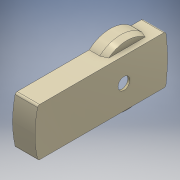
# Autodesk Inventor part: ET9
Saved by Autodesk Inventor 2016 (Build 200138000, 138)
## iProperties
Created: 2016-03-20
Part Number: ET9
Material: Genérico
Document SubType Name: Modeling
Designer: Usuario1
Density: 1 g/cm^3
Appearance: Valor por defecto
Author: Usuario1
Autodesk Inventor part; units mm, degrees
ref_plane "YZ Plane" through (0, 0, 0) normal (1, 0, 0) x (0, 1, 0)
ref_plane "XZ Plane" through (0, 0, 0) normal (0, 1, 0) x (-1, 0, 0)
ref_plane "XY Plane" through (0, 0, 0) normal (0, 0, 1) x (1, 0, 0)
sketch "Boceto1" plane through (0, 0, 0) normal (1, 0, 0) x (0, 1, 0)
  arc A0 (0.0357, 0.1637) -> (0.0357, -3.0114) centre (6.9261, -1.4239) ccw
  arc A1 (0.0357, -3.0114) -> (0.1818, -3.1278) centre (0.1818, -2.9778) ccw
  arc A2 (0.1818, 0.28) -> (0.0357, 0.1637) centre (0.1818, 0.13) ccw
  arc A3 (9.1854, -2.9976) -> (9.1854, 0.1498) centre (-2.6213, -1.4239) ccw
  arc A4 (9.0368, -3.1278) -> (9.1854, -2.9976) centre (9.0368, -2.9778) ccw
  arc A5 (9.1854, 0.1498) -> (9.0368, 0.28) centre (9.0368, 0.13) ccw
  line L0 (9.0368, 0.28) -> (8.2953, 0.28)
  line L1 (9.0368, -3.1278) -> (8.2953, -3.1278)
  line L2 (5.3121, 0.28) -> (0.1818, 0.28)
  line L3 (0.1818, -3.1278) -> (5.3121, -3.1278)
  arc A6 (8.2953, 0.28) -> (5.3121, 0.28) centre (6.8037, -1.4239) ccw
  arc A7 (5.3121, -3.1278) -> (8.2953, -3.1278) centre (6.8037, -1.4239) ccw
  arc A8 (9.0368, -2.9778) -> (9.0368, 0.13) centre (-2.6213, -1.4239) ccw
  line L4 (9.0368, -2.9778) -> (8.2378, -2.9778)
  arc A9 (5.3695, -2.9778) -> (8.2378, -2.9778) centre (6.8037, -1.4239) ccw
  line L5 (5.3695, -2.9778) -> (0.1818, -2.9778)
  arc A10 (0.1818, 0.13) -> (0.1818, -2.9778) centre (6.9261, -1.4239) ccw
  line L6 (0.1818, 0.13) -> (5.3695, 0.13)
  arc A11 (8.2378, 0.13) -> (5.3695, 0.13) centre (6.8037, -1.4239) ccw
  line L7 (8.2378, 0.13) -> (9.0368, 0.13)
  point P0 (0, 0)
  dimension "d0" = 0.15
  constraints: 24 point on circle, 16 end point, 12 centre point, 7 other
  measures "d0" radial gap between concentric circles of A3 A8
extrude "Extrusión1" add sketch "Boceto1" along normal blind 0.45
sketch "Boceto2" plane through (0.45, 0, 0) normal (1, 0, 0) x (0, 0, -1)
  line L0 (2.9778, 9.0368) -> (2.9778, 8.2378) projected
  arc A0 (2.9778, 5.3695) -> (2.9778, 8.2378) centre (1.4239, 6.8037) ccw projected
  line L1 (2.9778, 5.3695) -> (2.9778, 0.1818) projected
  arc A1 (-0.13, 0.1818) -> (2.9778, 0.1818) centre (1.4239, 6.9261) ccw projected
  line L2 (-0.13, 0.1818) -> (-0.13, 5.3695) projected
  arc A2 (-0.13, 8.2378) -> (-0.13, 5.3695) centre (1.4239, 6.8037) ccw projected
  line L3 (-0.13, 8.2378) -> (-0.13, 9.0368) projected
  arc A3 (2.9778, 9.0368) -> (-0.13, 9.0368) centre (1.4239, -2.6213) ccw projected
  arc A4 (-0.1637, 0.0357) -> (3.0114, 0.0357) centre (1.4239, 6.9261) ccw projected
  arc A5 (3.0114, 0.0357) -> (3.1278, 0.1818) centre (2.9778, 0.1818) ccw projected
  line L4 (3.1278, 0.1818) -> (3.1278, 5.3121) projected
  arc A6 (3.1278, 5.3121) -> (3.1278, 8.2953) centre (1.4239, 6.8037) ccw projected
  line L5 (3.1278, 8.2953) -> (3.1278, 9.0368) projected
  arc A7 (3.1278, 9.0368) -> (2.9976, 9.1854) centre (2.9778, 9.0368) ccw projected
  arc A8 (2.9976, 9.1854) -> (-0.1498, 9.1854) centre (1.4239, -2.6213) ccw projected
  arc A9 (-0.1498, 9.1854) -> (-0.28, 9.0368) centre (-0.13, 9.0368) ccw projected
  line L6 (-0.28, 9.0368) -> (-0.28, 8.2953) projected
  arc A10 (-0.28, 8.2953) -> (-0.28, 5.3121) centre (1.4239, 6.8037) ccw projected
  line L7 (-0.28, 5.3121) -> (-0.28, 0.1818) projected
  arc A11 (-0.28, 0.1818) -> (-0.1637, 0.0357) centre (-0.13, 0.1818) ccw projected
  line L8 (-0.13, 8.2378) -> (-0.13, 5.3695)
  arc A12 (2.9778, 5.3695) -> (2.9778, 8.2378) centre (1.4239, 6.8037) ccw projected
  line L9 (2.9778, 5.3695) -> (2.9778, 8.2378)
  point P0 (0, 0)
  constraints: 4 end point, 2 vertical
extrude "Extrusión2" add sketch "Boceto2" against normal blind 0.35 contours A0 L9 | L8 A2
chamfer "Chaflán1" distance 0.45 angle 15 1 edges at (0.45, 6.8037, -3.6884) measured on face at (0.35, 6.8037, -3.6884)
chamfer "Chaflán2" distance 0.45 angle 15 1 edges at (0.45, 6.8037, 0.8406) measured on face at (0.35, 6.8037, 0.8406)
sketch "Boceto3" plane through (0.45, 0, 0) normal (1, 0, 0) x (0, 0, -1)
  line L0 (-0.28, 0.1818) -> (-0.28, 5.5024) projected
  arc A0 (-0.28, 0.1818) -> (-0.1637, 0.0357) centre (-0.13, 0.1818) ccw projected
  arc A1 (-0.1637, 0.0357) -> (3.0114, 0.0357) centre (1.4239, 6.9261) ccw projected
  arc A2 (3.0114, 0.0357) -> (3.1278, 0.1818) centre (2.9778, 0.1818) ccw projected
  line L1 (3.1278, 0.1818) -> (3.1278, 5.5024) projected
  arc A3 (3.1278, 5.5024) -> (3.1278, 8.1049) centre (1.4239, 6.8037) ccw projected
  line L2 (3.1278, 9.0368) -> (3.1278, 8.1049) projected
  arc A4 (3.1278, 9.0368) -> (2.9976, 9.1854) centre (2.9778, 9.0368) ccw projected
  arc A5 (2.9976, 9.1854) -> (-0.1498, 9.1854) centre (1.4239, -2.6213) ccw projected
  arc A6 (-0.1498, 9.1854) -> (-0.28, 9.0368) centre (-0.13, 9.0368) ccw projected
  line L3 (-0.28, 9.0368) -> (-0.28, 8.1049) projected
  arc A7 (-0.28, 8.1049) -> (-0.28, 5.5024) centre (1.4239, 6.8037) ccw projected
  line L4 (2.9778, 9.0368) -> (2.9778, 0.1818) projected
  arc A8 (-0.13, 0.1818) -> (2.9778, 0.1818) centre (1.4239, 6.9261) ccw projected
  line L5 (-0.13, 0.1818) -> (-0.13, 9.0368) projected
  arc A9 (2.9778, 9.0368) -> (-0.13, 9.0368) centre (1.4239, -2.6213) ccw projected
  line L6 (-0.28, 8.1049) -> (-0.28, 5.5024)
  line L7 (3.1278, 8.1049) -> (3.1278, 5.5024)
  point P0 (0, 0)
  constraints: 4 end point, 1 parallel, 1 vertical
extrude "Extrusión3" add sketch "Boceto3" along normal blind 0.4 contours L0 L6 L3 A6 A5 A4 L2 L7 L1 A2 A1 A0
sketch "Boceto4" plane through (0.85, 0, 0) normal (1, 0, 0) x (0, 0, -1)
  arc A0 (-0.13, 0.1818) -> (2.9778, 0.1818) centre (1.4239, 6.9261) ccw projected
  line L0 (-0.13, 0.1818) -> (-0.13, 9.0368) projected
  arc A1 (2.9778, 9.0368) -> (-0.13, 9.0368) centre (1.4239, -2.6213) ccw projected
  line L1 (2.9778, 9.0368) -> (2.9778, 0.1818) projected
  line L2 (-0.28, 9.0368) -> (-0.28, 0.1818) projected
  arc A2 (-0.28, 0.1818) -> (-0.1637, 0.0357) centre (-0.13, 0.1818) ccw projected
  arc A3 (-0.1637, 0.0357) -> (3.0114, 0.0357) centre (1.4239, 6.9261) ccw projected
  arc A4 (3.0114, 0.0357) -> (3.1278, 0.1818) centre (2.9778, 0.1818) ccw projected
  line L3 (3.1278, 0.1818) -> (3.1278, 9.0368) projected
  arc A5 (3.1278, 9.0368) -> (2.9976, 9.1854) centre (2.9778, 9.0368) ccw projected
  arc A6 (2.9976, 9.1854) -> (-0.1498, 9.1854) centre (1.4239, -2.6213) ccw projected
  arc A7 (-0.1498, 9.1854) -> (-0.28, 9.0368) centre (-0.13, 9.0368) ccw projected
  point P0 (0, 0)
extrude "Extrusión4" add sketch "Boceto4" against normal blind 0.15 contours L0 A1 L1 A0
sketch "Boceto5" plane through (0, 0, 0) normal (-1, 0, 0) x (0, 0, 1)
  line L0 (-2.9778, 8.2378) -> (-2.9778, 9.0368) projected
  arc A0 (0.13, 9.0368) -> (-2.9778, 9.0368) centre (-1.4239, -2.6213) ccw projected
  line L1 (0.13, 9.0368) -> (0.13, 8.2378) projected
  arc A1 (0.13, 5.3695) -> (0.13, 8.2378) centre (-1.4239, 6.8037) ccw projected
  line L2 (0.13, 5.3695) -> (0.13, 0.1818) projected
  arc A2 (-2.9778, 0.1818) -> (0.13, 0.1818) centre (-1.4239, 6.9261) ccw projected
  line L3 (-2.9778, 0.1818) -> (-2.9778, 5.3695) projected
  arc A3 (-2.9778, 8.2378) -> (-2.9778, 5.3695) centre (-1.4239, 6.8037) ccw projected
  arc A4 (-3.0114, 0.0357) -> (0.1637, 0.0357) centre (-1.4239, 6.9261) ccw projected
  arc A5 (0.1637, 0.0357) -> (0.28, 0.1818) centre (0.13, 0.1818) ccw projected
  line L4 (0.28, 5.3121) -> (0.28, 0.1818) projected
  arc A6 (0.28, 5.3121) -> (0.28, 8.2953) centre (-1.4239, 6.8037) ccw projected
  line L5 (0.28, 9.0368) -> (0.28, 8.2953) projected
  arc A7 (0.28, 9.0368) -> (0.1498, 9.1854) centre (0.13, 9.0368) ccw projected
  arc A8 (0.1498, 9.1854) -> (-2.9976, 9.1854) centre (-1.4239, -2.6213) ccw projected
  arc A9 (-2.9976, 9.1854) -> (-3.1278, 9.0368) centre (-2.9778, 9.0368) ccw projected
  line L6 (-3.1278, 8.2953) -> (-3.1278, 9.0368) projected
  arc A10 (-3.1278, 8.2953) -> (-3.1278, 5.3121) centre (-1.4239, 6.8037) ccw projected
  line L7 (-3.1278, 0.1818) -> (-3.1278, 5.3121) projected
  arc A11 (-3.1278, 0.1818) -> (-3.0114, 0.0357) centre (-2.9778, 0.1818) ccw projected
  arc A12 (-3.0114, 0.0357) -> (0.1637, 0.0357) centre (-1.4239, 6.9261) ccw
  arc A13 (0.1637, 0.0357) -> (0.28, 0.1818) centre (0.13, 0.1818) ccw
  arc A14 (-3.1278, 0.1818) -> (-3.0114, 0.0357) centre (-2.9778, 0.1818) ccw
  circle A15 centre (-1.4239, 6.8037) radius 2.0393
  circle A16 centre (-2.9794, 4.0685) radius 0.092
  arc A17 (0.1498, 9.1854) -> (-2.9976, 9.1854) centre (-1.4239, -2.6213) ccw
  arc A18 (0.28, 9.0368) -> (0.1498, 9.1854) centre (0.13, 9.0368) ccw
  arc A19 (-2.9976, 9.1854) -> (-3.1278, 9.0368) centre (-2.9778, 9.0368) ccw
  line L8 (-3.1278, 3.94) -> (-2.9678, 3.94)
  arc A20 (-2.9678, 3.94) -> (-2.8478, 4.06) centre (-2.9678, 4.06) ccw
  line L9 (-2.8478, 4.06) -> (-2.8478, 4.0786)
  arc A21 (-2.8478, 4.0786) -> (-2.9678, 4.1986) centre (-2.9678, 4.0786) ccw
  line L10 (-2.9678, 4.1986) -> (-3.1278, 4.1986)
  circle A22 centre (-2.9778, 9.0368) radius 0.092
  line L11 (-3.1278, 8.9082) -> (-2.9678, 8.9082)
  line L12 (-2.8478, 9.2044) -> (-2.8478, 9.0282)
  arc A23 (-2.9678, 8.9082) -> (-2.8478, 9.0282) centre (-2.9678, 9.0282) ccw
  circle A24 centre (-2.9778, 0.1818) radius 0.092
  line L13 (-3.1278, 0.3104) -> (-2.9678, 0.3104)
  line L14 (-2.8478, 0) -> (-2.8478, 0.1904)
  arc A25 (-2.8478, 0.1904) -> (-2.9678, 0.3104) centre (-2.9678, 0.1904) ccw
  circle A26 centre (0.1317, 4.0685) radius 0.092
  line L15 (0.28, 3.94) -> (0.12, 3.94)
  arc A27 (0, 4.06) -> (0.12, 3.94) centre (0.12, 4.06) ccw
  line L16 (0, 4.06) -> (0, 4.0786)
  arc A28 (0.12, 4.1986) -> (0, 4.0786) centre (0.12, 4.0786) ccw
  line L17 (0.12, 4.1986) -> (0.28, 4.1986)
  circle A29 centre (0.13, 9.0368) radius 0.092
  line L18 (0.28, 8.9082) -> (0.12, 8.9082)
  line L19 (0, 9.2044) -> (0, 9.0282)
  arc A30 (0, 9.0282) -> (0.12, 8.9082) centre (0.12, 9.0282) ccw
  circle A31 centre (0.13, 0.1818) radius 0.092
  line L20 (0.28, 0.3104) -> (0.12, 0.3104)
  line L21 (0, 0) -> (0, 0.1904)
  arc A32 (0.12, 0.3104) -> (0, 0.1904) centre (0.12, 0.1904) ccw
  line L22 (-3.1278, 9.0368) -> (-3.1278, 8.2953)
  line L23 (0.28, 9.0368) -> (0.28, 8.2953)
  line L24 (-3.1278, 5.3121) -> (-3.1278, 0.1818)
  line L25 (0.28, 0.1818) -> (0.28, 5.3121)
  arc A33 (-3.1278, 8.2953) -> (-3.1278, 5.3121) centre (-1.4239, 6.8037) ccw
  arc A34 (0.28, 5.3121) -> (0.28, 8.2953) centre (-1.4239, 6.8037) ccw
  point P0 (0, 0)
  constraints: 36 end point, 36 point on circle, 23 centre point, 8 point on line
extrude "Extrusión5" add sketch "Boceto5" against normal blind 0.75 contours L11 L6 A9 A8 L12 A0 A22 L0 | L0 A22 A0 L12 A23 L11 | A22 A0 L0 | L0 A0 A22 | L10 A21 L9 A20 L8 L3 A16 | L3 A16 L8 L7 L10 | A16 L3 | L3 A16 | L19 A8 A7 L5 L18 L1 A29 A0 | A0 A29 L1 L18 A30 L19 | L13 L3 A24 A2 L14 A4 A11 L7 | A29 L1 A0 | A0 L1 A29 | L13 A25 L14 A2 A24 L3 | A24 A2 L3 | L3 A2 A24 | L21 A2 A31 L2 L20 L4 A5 A4 | L21 A32 L20 L2 A31 A2 | L17 L4 L15 L2 A26 | L2 A26 L15 A27 L16 A28 L17 | A31 L2 A2 | A2 L2 A31 | A26 L2 | L2 A26
sketch "Boceto6" plane through (0.1, 0, 0) normal (-1, 0, 0) x (0, 0, 1)
  line L0 (-2.9778, 5.3695) -> (-2.9778, 8.2378) projected
  arc A0 (-2.9778, 8.2378) -> (-2.9778, 5.3695) centre (-1.4239, 6.8037) ccw projected
  line L1 (0.13, 8.2378) -> (0.13, 5.3695) projected
  arc A1 (0.13, 5.3695) -> (0.13, 8.2378) centre (-1.4239, 6.8037) ccw projected
  point P0 (0, 0)
extrude "Extrusión6" add sketch "Boceto6" along normal blind 0.1
sketch "Boceto7" plane through (0, 0, 0) normal (-1, 0, 0) x (0, 0, 1)
  arc A0 (-2.8478, 0.1532) -> (0, 0.1532) centre (-1.4239, 6.9261) ccw projected
  line L0 (-2.8478, 0.1532) -> (-2.8478, 0.1904) projected
  arc A1 (-2.8478, 0.1904) -> (-2.9678, 0.3104) centre (-2.9678, 0.1904) ccw projected
  line L1 (-2.9678, 0.3104) -> (-2.9778, 0.3104) projected
  line L2 (-2.9778, 0.3104) -> (-2.9778, 3.94) projected
  line L3 (-2.9778, 3.94) -> (-2.9678, 3.94) projected
  arc A2 (-2.9678, 3.94) -> (-2.8478, 4.06) centre (-2.9678, 4.06) ccw projected
  line L4 (-2.8478, 4.06) -> (-2.8478, 4.0786) projected
  arc A3 (-2.8478, 4.0786) -> (-2.9678, 4.1986) centre (-2.9678, 4.0786) ccw projected
  line L5 (-2.9678, 4.1986) -> (-2.9778, 4.1986) projected
  line L6 (-2.9778, 4.1986) -> (-2.9778, 8.9082) projected
  line L7 (-2.9778, 8.9082) -> (-2.9678, 8.9082) projected
  arc A4 (-2.9678, 8.9082) -> (-2.8478, 9.0282) centre (-2.9678, 9.0282) ccw projected
  line L8 (-2.8478, 9.0282) -> (-2.8478, 9.0533) projected
  arc A5 (0, 9.0533) -> (-2.8478, 9.0533) centre (-1.4239, -2.6213) ccw projected
  line L9 (0, 9.0533) -> (0, 9.0282) projected
  arc A6 (0, 9.0282) -> (0.12, 8.9082) centre (0.12, 9.0282) ccw projected
  line L10 (0.12, 8.9082) -> (0.13, 8.9082) projected
  line L11 (0.13, 8.9082) -> (0.13, 4.1986) projected
  line L12 (0.13, 4.1986) -> (0.12, 4.1986) projected
  arc A7 (0.12, 4.1986) -> (0, 4.0786) centre (0.12, 4.0786) ccw projected
  line L13 (0, 4.0786) -> (0, 4.06) projected
  arc A8 (0, 4.06) -> (0.12, 3.94) centre (0.12, 4.06) ccw projected
  line L14 (0.12, 3.94) -> (0.13, 3.94) projected
  line L15 (0.13, 3.94) -> (0.13, 0.3104) projected
  line L16 (0.13, 0.3104) -> (0.12, 0.3104) projected
  arc A9 (0.12, 0.3104) -> (0, 0.1904) centre (0.12, 0.1904) ccw projected
  line L17 (0, 0.1904) -> (0, 0.1532) projected
  arc A10 (-3.0114, 0.0357) -> (0.1637, 0.0357) centre (-1.4239, 6.9261) ccw projected
  arc A11 (0.1637, 0.0357) -> (0.28, 0.1818) centre (0.13, 0.1818) ccw projected
  line L18 (0.28, 5.3121) -> (0.28, 0.1818) projected
  arc A12 (0.28, 5.3121) -> (0.28, 8.2953) centre (-1.4239, 6.8037) ccw projected
  line L19 (0.28, 9.0368) -> (0.28, 8.2953) projected
  arc A13 (0.28, 9.0368) -> (0.1498, 9.1854) centre (0.13, 9.0368) ccw projected
  arc A14 (0.1498, 9.1854) -> (-2.9976, 9.1854) centre (-1.4239, -2.6213) ccw projected
  arc A15 (-2.9976, 9.1854) -> (-3.1278, 9.0368) centre (-2.9778, 9.0368) ccw projected
  line L20 (-3.1278, 8.2953) -> (-3.1278, 9.0368) projected
  arc A16 (-3.1278, 8.2953) -> (-3.1278, 5.3121) centre (-1.4239, 6.8037) ccw projected
  line L21 (-3.1278, 0.1818) -> (-3.1278, 5.3121) projected
  arc A17 (-3.1278, 0.1818) -> (-3.0114, 0.0357) centre (-2.9778, 0.1818) ccw projected
  line L22 (0.28, 8.2953) -> (0.28, 5.3121)
  line L23 (-3.1278, 8.2953) -> (-3.1278, 9.0368) projected
  line L24 (-3.1278, 5.3121) -> (-3.1278, 8.2953)
  point P0 (0, 0)
  constraints: 4 end point, 1 collinear, 1 vertical
extrude "Extrusión7" add sketch "Boceto7" along normal blind 0.75 contours A17 L21 L24 L20 A15 A14 A13 L19 L22 L18 A11 A10
sketch "Boceto8" plane through (0, 0, 0) normal (-1, 0, 0) x (0, 0, 1)
  arc A0 (-3.1278, 8.1049) -> (-3.1278, 5.5024) centre (-1.4239, 6.8037) ccw projected
  arc A1 (-3.1278, 8.2953) -> (-3.1278, 5.3121) centre (-1.4239, 6.8037) ccw projected
  arc A2 (0.28, 5.5024) -> (0.28, 8.1049) centre (-1.4239, 6.8037) ccw projected
  arc A3 (0.28, 5.3121) -> (0.28, 8.2953) centre (-1.4239, 6.8037) ccw projected
  line L0 (-3.1278, 9.0368) -> (-3.1278, 0.1818) projected
  line L1 (0.28, 0.1818) -> (0.28, 9.0368) projected
  point P0 (0, 0)
extrude "Extrusión8" add sketch "Boceto8" along normal blind 0.75 contours A0 L0 A1 | A2 L1 A3
sketch "Boceto9" plane through (-0.75, 0, 0) normal (-1, 0, 0) x (0, 0, 1)
  arc A0 (0.28, 5.5024) -> (0.28, 8.1049) centre (-1.4239, 6.8037) ccw projected
  line L0 (0.28, 5.5024) -> (0.13, 5.5024)
  line L1 (0.13, 8.9082) -> (0.13, 4.1986) projected
  line L2 (0.28, 5.5024) -> (0.13, 5.5024)
  line L3 (-3.1278, 5.3121) -> (-3.1278, 0.1818) projected
  arc A1 (-3.1278, 0.1818) -> (-3.0114, 0.0357) centre (-2.9778, 0.1818) ccw projected
  arc A2 (-3.0114, 0.0357) -> (0.1637, 0.0357) centre (-1.4239, 6.9261) ccw projected
  arc A3 (0.1637, 0.0357) -> (0.28, 0.1818) centre (0.13, 0.1818) ccw projected
  line L4 (0.28, 0.1818) -> (0.28, 5.3121) projected
  arc A4 (0.28, 5.3121) -> (0.28, 8.2953) centre (-1.4239, 6.8037) ccw projected
  line L5 (0.28, 8.2953) -> (0.28, 9.0368) projected
  arc A5 (0.28, 9.0368) -> (0.1498, 9.1854) centre (0.13, 9.0368) ccw projected
  arc A6 (0.1498, 9.1854) -> (-2.9976, 9.1854) centre (-1.4239, -2.6213) ccw projected
  arc A7 (-2.9976, 9.1854) -> (-3.1278, 9.0368) centre (-2.9778, 9.0368) ccw projected
  line L6 (-3.1278, 9.0368) -> (-3.1278, 8.2953) projected
  arc A8 (-3.1278, 8.2953) -> (-3.1278, 5.3121) centre (-1.4239, 6.8037) ccw projected
  arc A9 (-3.1278, 8.1049) -> (-3.1278, 5.5024) centre (-1.4239, 6.8037) ccw projected
  line L7 (-3.1278, 8.1049) -> (-3.1278, 5.5024) projected
  line L8 (-2.8478, 0.1532) -> (-2.8478, 0.1904) projected
  arc A10 (-2.8478, 0.1904) -> (-2.9678, 0.3104) centre (-2.9678, 0.1904) ccw projected
  line L9 (-2.9678, 0.3104) -> (-2.9778, 0.3104) projected
  line L10 (-2.9778, 0.3104) -> (-2.9778, 3.94) projected
  line L11 (-2.9778, 3.94) -> (-2.9678, 3.94) projected
  arc A11 (-2.9678, 3.94) -> (-2.8478, 4.06) centre (-2.9678, 4.06) ccw projected
  line L12 (-2.8478, 4.06) -> (-2.8478, 4.0786) projected
  arc A12 (-2.8478, 4.0786) -> (-2.9678, 4.1986) centre (-2.9678, 4.0786) ccw projected
  line L13 (-2.9678, 4.1986) -> (-2.9778, 4.1986) projected
  line L14 (-2.9778, 4.1986) -> (-2.9778, 8.9082) projected
  line L15 (-2.9778, 8.9082) -> (-2.9678, 8.9082) projected
  arc A13 (-2.9678, 8.9082) -> (-2.8478, 9.0282) centre (-2.9678, 9.0282) ccw projected
  line L16 (-2.8478, 9.0282) -> (-2.8478, 9.0533) projected
  arc A14 (0, 9.0533) -> (-2.8478, 9.0533) centre (-1.4239, -2.6213) ccw projected
  line L17 (0, 9.0533) -> (0, 9.0282) projected
  arc A15 (0, 9.0282) -> (0.12, 8.9082) centre (0.12, 9.0282) ccw projected
  line L18 (0.12, 8.9082) -> (0.13, 8.9082) projected
  line L19 (0.13, 8.9082) -> (0.13, 4.1986) projected
  line L20 (0.13, 4.1986) -> (0.12, 4.1986) projected
  arc A16 (0.12, 4.1986) -> (0, 4.0786) centre (0.12, 4.0786) ccw projected
  line L21 (0, 4.0786) -> (0, 4.06) projected
  arc A17 (0, 4.06) -> (0.12, 3.94) centre (0.12, 4.06) ccw projected
  line L22 (0.12, 3.94) -> (0.13, 3.94) projected
  line L23 (0.13, 3.94) -> (0.13, 0.3104) projected
  line L24 (0.13, 0.3104) -> (0.12, 0.3104) projected
  arc A18 (0.12, 0.3104) -> (0, 0.1904) centre (0.12, 0.1904) ccw projected
  line L25 (0, 0.1904) -> (0, 0.1532) projected
  arc A19 (-2.8478, 0.1532) -> (0, 0.1532) centre (-1.4239, 6.9261) ccw projected
  arc A20 (0.28, 5.5024) -> (0.28, 8.1049) centre (-1.4239, 6.8037) ccw projected
  line L26 (0.28, 5.5024) -> (0.28, 8.1049) projected
  line L27 (0.28, 8.1049) -> (0.13, 8.1049)
  line L28 (-3.1278, 8.1049) -> (-2.9778, 8.1049)
  line L29 (-3.1278, 8.1049) -> (-3.1278, 5.5024) projected
  line L30 (-3.1278, 5.5024) -> (-2.9778, 5.5024)
  line L31 (-2.9778, 4.1986) -> (-2.9778, 8.9082) projected
  line L32 (-3.1278, 5.5024) -> (-3.1278, 8.1049)
  line L33 (-3.1278, 8.1049) -> (-2.9778, 8.1049)
  line L34 (-2.9778, 8.1049) -> (-2.9778, 5.5024)
  line L35 (0.28, 5.5024) -> (0.28, 8.1049)
  line L36 (0.28, 9.0368) -> (0.28, 0.1818) projected
  line L37 (0.13, 5.5024) -> (0.13, 8.1049)
  line L38 (-2.9778, 5.5024) -> (-3.1278, 5.5024)
  line L39 (-3.1278, 5.5024) -> (-3.1278, 8.1049)
  line L40 (-3.1278, 8.1049) -> (-2.9778, 8.1049)
  line L41 (-2.9778, 8.1049) -> (-2.9778, 5.5024)
  line L42 (0.28, 5.5024) -> (0.13, 5.5024)
  line L43 (0.13, 5.5024) -> (0.13, 8.1049)
  line L44 (0.13, 8.1049) -> (0.28, 8.1049)
  line L45 (0.28, 8.1049) -> (0.28, 5.5024)
  point P0 (0, 0)
  constraints: 36 end point, 6 point on line, 5 parallel, 5 perpendicular, 4 collinear, 3 horizontal
extrude "Extrusión9" cut sketch "Boceto9" against normal blind 0.75 contours L0 L1 L27 L26 | L14 L30 L7 L28
sketch "Boceto10" plane through (0.85, 0, 0) normal (1, 0, 0) x (0, 0, -1)
  line L0 (-0.28, 9.0368) -> (-0.28, 0.1818) projected
  arc A0 (-0.28, 0.1818) -> (-0.1637, 0.0357) centre (-0.13, 0.1818) ccw projected
  arc A1 (-0.1637, 0.0357) -> (3.0114, 0.0357) centre (1.4239, 6.9261) ccw projected
  arc A2 (3.0114, 0.0357) -> (3.1278, 0.1818) centre (2.9778, 0.1818) ccw projected
  line L1 (3.1278, 0.1818) -> (3.1278, 9.0368) projected
  arc A3 (3.1278, 9.0368) -> (2.9976, 9.1854) centre (2.9778, 9.0368) ccw projected
  arc A4 (2.9976, 9.1854) -> (-0.1498, 9.1854) centre (1.4239, -2.6213) ccw projected
  arc A5 (-0.1498, 9.1854) -> (-0.28, 9.0368) centre (-0.13, 9.0368) ccw projected
  arc A6 (2.9976, 9.1854) -> (-0.1498, 9.1854) centre (1.4239, -2.6213) ccw projected
  circle A7 centre (1.4239, 6.1899) radius 0.225
  circle A8 centre (1.4239, 6.1899) radius 0.425
  point P0 (0, 0)
  dimension "d26" = 0.45
  dimension "d29" = 0.85
  constraints: 2 centre point, 1 coincident
  measures "d26" diameter of A7
  measures "d29" diameter of A8
extrude "Extrusión10" cut sketch "Boceto10" against normal blind 0.5 contours A7 | A8
